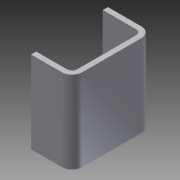
# Autodesk Inventor part: new support for PG-71
Saved by Autodesk Inventor 2013 (Build 170138000, 138)
## iProperties
Created: 2013-02-02
Part Number: new support for PG-71
Material: Aluminum 6061
Document SubType Name: Sheet Metal
Designer: aslane
Density: 1 g/cm^3
Sheet Metal Rule: Default
Author: aslane
Autodesk Inventor part; units mm, degrees
ref_plane "YZ Plane" through (0, 0, 0) normal (1, 0, 0) x (0, 1, 0)
ref_plane "XZ Plane" through (0, 0, 0) normal (0, 1, 0) x (-1, 0, 0)
ref_plane "XY Plane" through (0, 0, 0) normal (0, 0, 1) x (1, 0, 0)
sketch "Sketch1" plane through (0, 0, 0) normal (0, 0, 1) x (1, 0, 0)
  line L0 (0, 0) -> (25.4, 0)
  line L1 (25.4, 0) -> (25.4, 50.8)
  line L2 (25.4, 50.8) -> (0, 50.8)
  line L3 (0, 50.8) -> (0, 0)
  line L4 (25.4, 0) -> (44.45, 0)
  line L5 (44.45, 0) -> (44.45, 50.8)
  line L6 (44.45, 50.8) -> (25.4, 50.8)
  dimension "d0" = 25.4
  dimension "d1" = 50.8
  dimension "d27" = 19.05
  measures "d0" distance of L0.start L0.end
  measures "d1" distance of L0.end L1.end
  measures "d27" distance of L0.end L4.end
extrude "Plate1" add sketch "Sketch1" along normal blind 3.175 contours L3 L2 L1 L0
sketch "Sketch2" plane through (22.225, 0, 3.175) normal (1, 0, 0) x (0, 1, 0)
  line L0 (50.8, 0) -> (0, 0)
  line L1 (0, 0) -> (0, -49.213)
  line L2 (0, -49.213) -> (50.8, -49.213)
  line L3 (50.8, -49.213) -> (50.8, 0)
  constraints: 6 end point, 1 horizontal, 1 perpendicular, 1 vertical
edge flange "Flange1" height 49.213 angle 90 thickness 3.175 bend radius 3.175 thickness toward (1, 0, 0) relief straight relief width 3.175 relief depth 1.5875 edges at (25.4, 25.4, 0) wall of the first edge with corners at (22.225, 50.8, 3.175) (22.225, 0, 3.175) (22.225, 0, -46.038) (22.225, 50.8, -46.038)
bend "Bend1"
corner "Corner1"
sketch "Sketch3" plane through (25.4, 0, -42.863) normal (0, 0, -1) x (-1, 0, 0)
  line L0 (0, 50.8) -> (0, 0)
  line L1 (0, 0) -> (25.4, 0)
  line L2 (25.4, 0) -> (25.4, 50.8)
  line L3 (25.4, 50.8) -> (0, 50.8)
  constraints: 6 end point, 1 horizontal, 1 perpendicular, 1 vertical
edge flange "Flange2" height 25.4 angle 90 thickness 3.175 bend radius 3.175 thickness toward (0, 0, -1) relief straight relief width 3.175 relief depth 1.5875 edges at (22.225, 25.4, -46.038) wall of the first edge with corners at (25.4, 50.8, -42.863) (25.4, 0, -42.863) (0, 0, -42.863) (0, 50.8, -42.863)
bend "Bend2"
corner "Corner2"
sketch "Sketch4" plane through (0, 0, -46.038) normal (-1, 0, 0) x (0, 0, 1)
  line L0 (0, 50.8) -> (0, 0) projected
  line L1 (3.175, 0) -> (0, 0) projected
  line L2 (3.175, 50.8) -> (3.175, 0) projected
  line L3 (3.175, 50.8) -> (0, 50.8) projected
  point P0 (46.038, 0)
extrude "Extrusion1" add sketch "Sketch4" along normal blind 14.3256
sketch "Sketch5" plane through (-14.3256, 0, -46.038) normal (-1, 0, 0) x (0, 0, 1)
  line L0 (0, 50.8) -> (0, 0) projected
  line L1 (0, 0) -> (3.175, 0) projected
  line L2 (3.175, 0) -> (3.175, 50.8) projected
  line L3 (3.175, 50.8) -> (0, 50.8) projected
  point P0 (46.038, 0)
extrude "Extrusion2" cut sketch "Sketch5" against normal blind 12.7
equation "\"d3\" = BendReliefWidth"
equation "\"d4\" = BendReliefDepth"
equation "\"d5\" = MinimumRemnant"
equation "\"d6\" = BendRadius"
equation "\"d10\" = CornerReliefSize"
equation "\"d11\" = GapSize"
equation "\"d12\" = JacobiRadiusSize"
equation "\"d13\" = BendReliefWidth"
equation "\"d14\" = BendReliefDepth"
equation "\"d15\" = MinimumRemnant"
equation "\"d16\" = BendRadius"
equation "\"d20\" = CornerReliefSize"
equation "\"d21\" = GapSize"
equation "\"d22\" = JacobiRadiusSize"
equation "\"BendRadius\" = Thickness"
equation "\"BendReliefWidth\" = Thickness"
equation "\"BendReliefDepth\" = 0.5 * Thickness"
equation "\"CornerReliefSize\" = 4 * Thickness"
equation "\"MinimumRemnant\" = 2 * Thickness"
equation "\"TransitionRadius\" = BendRadius"
equation "\"JacobiRadiusSize\" = BendRadius"
equation "\"GapSize\" = Thickness"
equation "\"d2\" = BendRadius"
equation "\"Thickness\" = 3.175"
body "Solid1"
